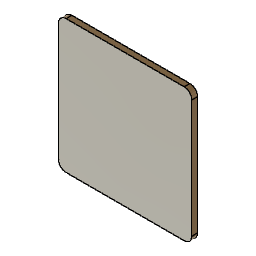
bottom_access_panel (Autodesk Fusion 360 design; units mm, degrees)
Autodesk Fusion 360 part; units mm, degrees
sketch "Top Access Panel" plane through (0, 0, 0) normal (0, 1, 0) x (1, 0, 0)
  line L0 (0, 0) -> (140, 0)
  line L1 (140, 0) -> (140, -140)
  line L2 (140, -140) -> (0, -140)
  line L3 (0, -140) -> (0, 0)
  dimension "d1" = 140
  dimension "d2" = 140
  constraint horizontal L0
  constraint vertical L1
  constraint horizontal L2
  constraint vertical L3
  constraint coincident L0.start L3.end
  measures "d1" distance of L0.start L0.end
  measures "d2" distance of L0.end L1.end
extrude "Extrude1" add sketch "Top Access Panel" along normal blind 6
fillet "Fillet1" radius 8 4 edges at (0, 3, 140) (140, 3, 140) (140, 3, 0) (0, 3, 0)
equation "mdfThickness = 6 mm" comment "Thickness of the MDF fibre board"
equation "d4 = mdfThickness"
equation "filletRadius = 8 mm" comment "Radius to use for fillets"
equation "d15 = filletRadius"
named bodies: "Bottom Access Panel"
